Autodesk Inventor part; units mm, degrees
(part 2 of 3)
  spline S130 degree 2 poles (57.6715, -7.9736) (57.2251, -7.5754) (56.7568, -7.4309) knots 0 0 0 1 1 1
  line L163 (56.7568, -7.4309) -> (56.735, -7.3434)
  spline S131 degree 2 poles (56.735, -7.3434) (56.8662, -7.2603) (56.9144, -7.1727) knots 0 0 0 1 1 1
  spline S132 degree 2 poles (56.9144, -7.1727) (57.0019, -7.024) (57.0019, -6.8139) knots 0 0 0 1 1 1
  line L164 (57.0019, -6.8139) -> (57.0019, -4.7133)
  line L165 (57.0019, -4.7133) -> (56.6649, -4.7133)
  line L166 (56.6649, -4.7133) -> (56.6649, -4.3107)
  line L167 (56.6649, -4.3107) -> (57.0019, -4.3107)
  line L168 (57.0019, -4.3107) -> (57.0019, -3.4443)
  spline S133 degree 2 poles (57.0019, -3.4443) (57.5402, -3.0767) (57.8159, -2.8272) knots 0 0 0 1 1 1
  line L169 (57.8159, -2.8272) -> (58.4985, -2.9979)
  line L170 (58.7611, -4.5383) -> (59.7589, -3.3042)
  line L171 (59.7589, -3.3042) -> (59.8639, -3.3042)
  line L172 (59.8639, -3.3042) -> (59.8289, -4.2932)
  line L173 (59.8289, -4.2932) -> (60.551, -4.2932)
  line L174 (60.551, -4.2932) -> (60.551, -4.6958)
  line L175 (60.551, -4.6958) -> (59.8289, -4.6958)
  line L176 (59.8289, -4.6958) -> (59.8289, -7.1159)
  line L177 (59.8289, -7.1159) -> (60.2315, -7.4134)
  line L178 (60.2315, -7.4134) -> (60.4634, -7.234)
  line L179 (60.4634, -7.234) -> (60.5553, -7.3434)
  line L180 (60.5553, -7.3434) -> (59.7633, -7.9736)
  spline S134 degree 2 poles (59.7633, -7.9736) (59.3563, -7.5622) (58.8486, -7.4134) knots 0 0 0 1 1 1
  line L181 (58.8486, -7.4134) -> (58.8486, -7.3434)
  spline S135 degree 2 poles (58.8486, -7.3434) (58.9931, -7.2471) (59.0368, -7.1421) knots 0 0 0 1 1 1
  spline S136 degree 2 poles (59.0368, -7.1421) (59.0981, -7.0108) (59.0981, -6.757) knots 0 0 0 1 1 1
  line L182 (59.0981, -6.757) -> (59.0981, -4.6958)
  line L183 (59.0981, -4.6958) -> (58.7611, -4.6958)
  line L184 (58.7611, -4.6958) -> (58.7611, -4.5383)
  point P0 (76.2, -5.7603)
  point P1 (0, 5.7603)
  constraints: 2 other
extrude "Extrusion5" add sketch "Sketch6" along normal blind 0.2286
sketch "Sketch7" plane through (-5.7603, -3.3257, 0) normal (-0.8660254, 0.5, 0) x (0, 0, 1)
  line L0 (0.5735, 1.7459) -> (40.1435, 1.7459) construction
  line L1 (40.1435, 1.7459) -> (40.1435, 0.1688) construction
  line L2 (40.1435, 0.1688) -> (0.5735, 0.1688) construction
  line L3 (0.5735, 0.1688) -> (0.5735, 1.7459) construction
  spline S0 degree 2 poles (2.0565, 0.9853) (2.0565, 0.867) (1.9917, 0.6457) (1.931, 0.5541) knots 0 0 0 1 2 2 2
  line L4 (1.931, 0.5541) -> (1.5728, 0.5541)
  line L5 (1.5728, 0.5541) -> (1.5512, 0.6529)
  spline S1 degree 2 poles (1.5512, 0.6529) (1.4936, 0.6045) (1.3978, 0.5469) (1.3145, 0.5469) knots 0 0 0 1 2 2 2
  spline S2 degree 2 poles (1.3145, 0.5469) (1.1838, 0.5469) (1.016, 0.7579) (1.016, 0.9576) knots 0 0 0 1 2 2 2
  spline S3 degree 2 poles (1.016, 0.9576) (1.016, 1.1582) (1.2219, 1.3816) (1.3546, 1.3816) knots 0 0 0 1 2 2 2
  spline S4 degree 2 poles (1.3546, 1.3816) (1.4164, 1.3816) (1.5049, 1.3507) (1.5502, 1.325) knots 0 0 0 1 2 2 2
  line L6 (1.5502, 1.325) -> (1.5502, 1.3661)
  line L7 (1.5502, 1.3661) -> (1.685, 1.3661)
  line L8 (1.685, 1.3661) -> (1.685, 0.6488)
  line L9 (1.685, 0.6488) -> (1.8785, 0.6488)
  spline S5 degree 2 poles (1.8785, 0.6488) (1.9114, 0.7095) (1.9392, 0.902) (1.9392, 0.9802) knots 0 0 0 1 2 2 2
  spline S6 degree 2 poles (1.9392, 0.9802) (1.9392, 1.2591) (1.6551, 1.5987) (1.3886, 1.5987) knots 0 0 0 1 2 2 2
  spline S7 degree 2 poles (1.3886, 1.5987) (1.1364, 1.5987) (0.8081, 1.2313) (0.8081, 0.9689) knots 0 0 0 1 2 2 2
  spline S8 degree 2 poles (0.8081, 0.9689) (0.8081, 0.6879) (1.1272, 0.339) (1.3845, 0.339) knots 0 0 0 1 2 2 2
  spline S9 degree 2 poles (1.3845, 0.339) (1.4534, 0.339) (1.6068, 0.3575) (1.6747, 0.3781) knots 0 0 0 1 2 2 2
  line L10 (1.6747, 0.3781) -> (1.6747, 0.2577)
  spline S10 degree 2 poles (1.6747, 0.2577) (1.6027, 0.2402) (1.4555, 0.2268) (1.3834, 0.2268) knots 0 0 0 1 2 2 2
  spline S11 degree 2 poles (1.3834, 0.2268) (1.0819, 0.2268) (0.6857, 0.6416) (0.6857, 0.9709) knots 0 0 0 1 2 2 2
  spline S12 degree 2 poles (0.6857, 0.9709) (0.6857, 1.2838) (1.0942, 1.714) (1.3876, 1.714) knots 0 0 0 1 2 2 2
  spline S13 degree 2 poles (1.3876, 1.714) (1.7015, 1.714) (2.0565, 1.3095) (2.0565, 0.9853) knots 0 0 0 1 2 2 2
  line L11 (1.5481, 0.7672) -> (1.5481, 1.2087)
  spline S14 degree 2 poles (1.5481, 1.2087) (1.5008, 1.2334) (1.4205, 1.255) (1.3762, 1.255) knots 0 0 0 1 2 2 2
  spline S15 degree 2 poles (1.3762, 1.255) (1.2795, 1.255) (1.1622, 1.1109) (1.1622, 0.9596) knots 0 0 0 1 2 2 2
  spline S16 degree 2 poles (1.1622, 0.9596) (1.1622, 0.8238) (1.2507, 0.6786) (1.3484, 0.6786) knots 0 0 0 1 2 2 2
  spline S17 degree 2 poles (1.3484, 0.6786) (1.3999, 0.6786) (1.5018, 0.728) (1.5481, 0.7672) knots 0 0 0 1 2 2 2
  line L12 (3.379, 0.4193) -> (3.2102, 0.4193)
  line L13 (3.2102, 0.4193) -> (3.2102, 1.5133)
  line L14 (3.2102, 1.5133) -> (2.8788, 0.7692)
  line L15 (2.8788, 0.7692) -> (2.7759, 0.7692)
  line L16 (2.7759, 0.7692) -> (2.4476, 1.5133)
  line L17 (2.4476, 1.5133) -> (2.4476, 0.4193)
  line L18 (2.4476, 0.4193) -> (2.2901, 0.4193)
  line L19 (2.2901, 0.4193) -> (2.2901, 1.6893)
  line L20 (2.2901, 1.6893) -> (2.5207, 1.6893)
  line L21 (2.5207, 1.6893) -> (2.8377, 0.9823)
  line L22 (2.8377, 0.9823) -> (3.1444, 1.6893)
  line L23 (3.1444, 1.6893) -> (3.379, 1.6893)
  line L24 (3.379, 1.6893) -> (3.379, 0.4193)
  line L25 (3.7876, 0.4193) -> (3.627, 0.4193)
  line L26 (3.627, 0.4193) -> (3.627, 1.3723)
  line L27 (3.627, 1.3723) -> (3.7876, 1.3723)
  line L28 (3.7876, 1.3723) -> (3.7876, 0.4193)
  line L29 (3.7989, 1.5308) -> (3.6167, 1.5308)
  line L30 (3.6167, 1.5308) -> (3.6167, 1.6975)
  line L31 (3.6167, 1.6975) -> (3.7989, 1.6975)
  line L32 (3.7989, 1.6975) -> (3.7989, 1.5308)
  spline S18 degree 2 poles (4.2806, 0.3967) (4.1848, 0.3967) (4.0192, 0.4481) (3.9646, 0.4769) knots 0 0 0 1 2 2 2
  line L33 (3.9646, 0.4769) -> (3.9646, 0.657)
  line L34 (3.9646, 0.657) -> (3.9728, 0.657)
  spline S19 degree 2 poles (3.9728, 0.657) (3.9934, 0.6406) (4.049, 0.6015) (4.0953, 0.5798) knots 0 0 0 1 2 2 2
  spline S20 degree 2 poles (4.0953, 0.5798) (4.1354, 0.5603) (4.2342, 0.5315) (4.2867, 0.5315) knots 0 0 0 1 2 2 2
  spline S21 degree 2 poles (4.2867, 0.5315) (4.3248, 0.5315) (4.4123, 0.549) (4.4329, 0.5634) knots 0 0 0 1 2 2 2
  spline S22 degree 2 poles (4.4329, 0.5634) (4.4627, 0.5829) (4.4895, 0.6272) (4.4895, 0.6725) knots 0 0 0 1 2 2 2
  spline S23 degree 2 poles (4.4895, 0.6725) (4.4895, 0.7291) (4.4277, 0.7877) (4.3485, 0.8073) knots 0 0 0 1 2 2 2
  spline S24 degree 2 poles (4.3485, 0.8073) (4.3176, 0.8145) (4.2188, 0.8351) (4.1766, 0.8464) knots 0 0 0 1 2 2 2
  spline S25 degree 2 poles (4.1766, 0.8464) (4.0675, 0.8783) (3.9687, 1.01) (3.9687, 1.1037) knots 0 0 0 1 2 2 2
  spline S26 degree 2 poles (3.9687, 1.1037) (3.9687, 1.2334) (4.1632, 1.395) (4.3238, 1.395) knots 0 0 0 1 2 2 2
  spline S27 degree 2 poles (4.3238, 1.395) (4.403, 1.395) (4.5636, 1.3558) (4.6181, 1.326) knots 0 0 0 1 2 2 2
  line L35 (4.6181, 1.326) -> (4.6181, 1.1541)
  line L36 (4.6181, 1.1541) -> (4.6099, 1.1541)
  spline S28 degree 2 poles (4.6099, 1.1541) (4.5481, 1.2035) (4.3979, 1.2601) (4.3207, 1.2601) knots 0 0 0 1 2 2 2
  spline S29 degree 2 poles (4.3207, 1.2601) (4.2415, 1.2601) (4.1324, 1.1932) (4.1324, 1.1263) knots 0 0 0 1 2 2 2
  spline S30 degree 2 poles (4.1324, 1.1263) (4.1324, 1.0656) (4.1972, 1.007) (4.2692, 0.9884) knots 0 0 0 1 2 2 2
  spline S31 degree 2 poles (4.2692, 0.9884) (4.3042, 0.9792) (4.3927, 0.9606) (4.4411, 0.9493) knots 0 0 0 1 2 2 2
  spline S32 degree 2 poles (4.4411, 0.9493) (4.5461, 0.9226) (4.6531, 0.8001) (4.6531, 0.6941) knots 0 0 0 1 2 2 2
  spline S33 degree 2 poles (4.6531, 0.6941) (4.6531, 0.6323) (4.6048, 0.5232) (4.5574, 0.4831) knots 0 0 0 1 2 2 2
  spline S34 degree 2 poles (4.5574, 0.4831) (4.507, 0.4409) (4.3783, 0.3967) (4.2806, 0.3967) knots 0 0 0 1 2 2 2
  spline S35 degree 2 poles (5.0596, 0.3967) (4.9639, 0.3967) (4.7982, 0.4481) (4.7437, 0.4769) knots 0 0 0 1 2 2 2
  line L37 (4.7437, 0.4769) -> (4.7437, 0.657)
  line L38 (4.7437, 0.657) -> (4.7519, 0.657)
  spline S36 degree 2 poles (4.7519, 0.657) (4.7725, 0.6406) (4.8281, 0.6015) (4.8744, 0.5798) knots 0 0 0 1 2 2 2
  spline S37 degree 2 poles (4.8744, 0.5798) (4.9145, 0.5603) (5.0133, 0.5315) (5.0658, 0.5315) knots 0 0 0 1 2 2 2
  spline S38 degree 2 poles (5.0658, 0.5315) (5.1039, 0.5315) (5.1914, 0.549) (5.212, 0.5634) knots 0 0 0 1 2 2 2
  spline S39 degree 2 poles (5.212, 0.5634) (5.2418, 0.5829) (5.2686, 0.6272) (5.2686, 0.6725) knots 0 0 0 1 2 2 2
  spline S40 degree 2 poles (5.2686, 0.6725) (5.2686, 0.7291) (5.2068, 0.7877) (5.1276, 0.8073) knots 0 0 0 1 2 2 2
  spline S41 degree 2 poles (5.1276, 0.8073) (5.0967, 0.8145) (4.9979, 0.8351) (4.9557, 0.8464) knots 0 0 0 1 2 2 2
  spline S42 degree 2 poles (4.9557, 0.8464) (4.8466, 0.8783) (4.7478, 1.01) (4.7478, 1.1037) knots 0 0 0 1 2 2 2
  spline S43 degree 2 poles (4.7478, 1.1037) (4.7478, 1.2334) (4.9423, 1.395) (5.1029, 1.395) knots 0 0 0 1 2 2 2
  spline S44 degree 2 poles (5.1029, 1.395) (5.1821, 1.395) (5.3427, 1.3558) (5.3972, 1.326) knots 0 0 0 1 2 2 2
  line L39 (5.3972, 1.326) -> (5.3972, 1.1541)
  line L40 (5.3972, 1.1541) -> (5.389, 1.1541)
  spline S45 degree 2 poles (5.389, 1.1541) (5.3272, 1.2035) (5.177, 1.2601) (5.0998, 1.2601) knots 0 0 0 1 2 2 2
  spline S46 degree 2 poles (5.0998, 1.2601) (5.0205, 1.2601) (4.9114, 1.1932) (4.9114, 1.1263) knots 0 0 0 1 2 2 2
  spline S47 degree 2 poles (4.9114, 1.1263) (4.9114, 1.0656) (4.9763, 1.007) (5.0483, 0.9884) knots 0 0 0 1 2 2 2
  spline S48 degree 2 poles (5.0483, 0.9884) (5.0833, 0.9792) (5.1718, 0.9606) (5.2202, 0.9493) knots 0 0 0 1 2 2 2
  spline S49 degree 2 poles (5.2202, 0.9493) (5.3252, 0.9226) (5.4322, 0.8001) (5.4322, 0.6941) knots 0 0 0 1 2 2 2
  spline S50 degree 2 poles (5.4322, 0.6941) (5.4322, 0.6323) (5.3838, 0.5232) (5.3365, 0.4831) knots 0 0 0 1 2 2 2
  spline S51 degree 2 poles (5.3365, 0.4831) (5.2861, 0.4409) (5.1574, 0.3967) (5.0596, 0.3967) knots 0 0 0 1 2 2 2
  line L41 (5.7451, 0.4193) -> (5.5845, 0.4193)
  line L42 (5.5845, 0.4193) -> (5.5845, 1.3723)
  line L43 (5.5845, 1.3723) -> (5.7451, 1.3723)
  line L44 (5.7451, 1.3723) -> (5.7451, 0.4193)
  line L45 (5.7564, 1.5308) -> (5.5742, 1.5308)
  line L46 (5.5742, 1.5308) -> (5.5742, 1.6975)
  line L47 (5.5742, 1.6975) -> (5.7564, 1.6975)
  line L48 (5.7564, 1.6975) -> (5.7564, 1.5308)
  spline S52 degree 2 poles (6.764, 0.8958) (6.764, 0.655) (6.5324, 0.3925) (6.3389, 0.3925) knots 0 0 0 1 2 2 2
  spline S53 degree 2 poles (6.3389, 0.3925) (6.1403, 0.3925) (5.9128, 0.6632) (5.9128, 0.8958) knots 0 0 0 1 2 2 2
  spline S54 degree 2 poles (5.9128, 0.8958) (5.9128, 1.1346) (6.1475, 1.3991) (6.3389, 1.3991) knots 0 0 0 1 2 2 2
  spline S55 degree 2 poles (6.3389, 1.3991) (6.5324, 1.3991) (6.764, 1.1356) (6.764, 0.8958) knots 0 0 0 1 2 2 2
  spline S56 degree 2 poles (6.5983, 0.8958) (6.5983, 1.0811) (6.4634, 1.2612) (6.3389, 1.2612) knots 0 0 0 1 2 2 2
  spline S57 degree 2 poles (6.3389, 1.2612) (6.2144, 1.2612) (6.0785, 1.0811) (6.0785, 0.8958) knots 0 0 0 1 2 2 2
  spline S58 degree 2 poles (6.0785, 0.8958) (6.0785, 0.7157) (6.2144, 0.5304) (6.3389, 0.5304) knots 0 0 0 1 2 2 2
  spline S59 degree 2 poles (6.3389, 0.5304) (6.4624, 0.5304) (6.5983, 0.7126) (6.5983, 0.8958) knots 0 0 0 1 2 2 2
  line L49 (7.6768, 0.4193) -> (7.5163, 0.4193)
  line L50 (7.5163, 0.4193) -> (7.5163, 0.9627)
  spline S60 degree 2 poles (7.5163, 0.9627) (7.5163, 1.0286) (7.5039, 1.1418) (7.4854, 1.1757) knots 0 0 0 1 2 2 2
  spline S61 degree 2 poles (7.4854, 1.1757) (7.4659, 1.2118) (7.3959, 1.2468) (7.3362, 1.2468) knots 0 0 0 1 2 2 2
  spline S62 degree 2 poles (7.3362, 1.2468) (7.2765, 1.2468) (7.1499, 1.1829) (7.0892, 1.1315) knots 0 0 0 1 2 2 2
  line L51 (7.0892, 1.1315) -> (7.0892, 0.4193)
  line L52 (7.0892, 0.4193) -> (6.9286, 0.4193)
  line L53 (6.9286, 0.4193) -> (6.9286, 1.3723)
  line L54 (6.9286, 1.3723) -> (7.0892, 1.3723)
  line L55 (7.0892, 1.3723) -> (7.0892, 1.2663)
  spline S63 degree 2 poles (7.0892, 1.2663) (7.1612, 1.3311) (7.3002, 1.3991) (7.3784, 1.3991) knots 0 0 0 1 2 2 2
  spline S64 degree 2 poles (7.3784, 1.3991) (7.5183, 1.3991) (7.6768, 1.2138) (7.6768, 1.0378) knots 0 0 0 1 2 2 2
  line L56 (7.6768, 1.0378) -> (7.6768, 0.4193)
  spline S65 degree 2 poles (8.8141, 0.3967) (8.6762, 0.3967) (8.4827, 0.4543) (8.3973, 0.4955) knots 0 0 0 1 2 2 2
  line L57 (8.3973, 0.4955) -> (8.3973, 0.7075)
  line L58 (8.3973, 0.7075) -> (8.4096, 0.7075)
  spline S66 degree 2 poles (8.4096, 0.7075) (8.493, 0.6292) (8.7039, 0.5428) (8.8017, 0.5428) knots 0 0 0 1 2 2 2
  spline S67 degree 2 poles (8.8017, 0.5428) (8.9417, 0.5428) (9.0847, 0.6591) (9.0847, 0.7548) knots 0 0 0 1 2 2 2
  spline S68 degree 2 poles (9.0847, 0.7548) (9.0847, 0.831) (9.0096, 0.9257) (8.9283, 0.9493) knots 0 0 0 1 2 2 2
  spline S69 degree 2 poles (8.9283, 0.9493) (8.8696, 0.9658) (8.7719, 0.9884) (8.6988, 1.007) knots 0 0 0 1 2 2 2
  spline S70 degree 2 poles (8.6988, 1.007) (8.6329, 1.0245) (8.529, 1.0769) (8.4889, 1.1191) knots 0 0 0 1 2 2 2
  spline S71 degree 2 poles (8.4889, 1.1191) (8.4497, 1.1613) (8.4065, 1.2745) (8.4065, 1.3486) knots 0 0 0 1 2 2 2
  spline S72 degree 2 poles (8.4065, 1.3486) (8.4065, 1.503) (8.6473, 1.7119) (8.8336, 1.7119) knots 0 0 0 1 2 2 2
  spline S73 degree 2 poles (8.8336, 1.7119) (8.9407, 1.7119) (9.13, 1.6697) (9.2113, 1.6296) knots 0 0 0 1 2 2 2
  line L59 (9.2113, 1.6296) -> (9.2113, 1.4279)
  line L60 (9.2113, 1.4279) -> (9.199, 1.4279)
  spline S74 degree 2 poles (9.199, 1.4279) (9.1383, 1.4835) (8.9489, 1.5658) (8.8449, 1.5658) knots 0 0 0 1 2 2 2
  spline S75 degree 2 poles (8.8449, 1.5658) (8.7276, 1.5658) (8.5825, 1.4557) (8.5825, 1.3661) knots 0 0 0 1 2 2 2
  spline S76 degree 2 poles (8.5825, 1.3661) (8.5825, 1.2859) (8.6679, 1.1901) (8.7482, 1.1685) knots 0 0 0 1 2 2 2
  spline S77 degree 2 poles (8.7482, 1.1685) (8.8017, 1.1541) (8.9571, 1.1171) (9.0086, 1.1016) knots 0 0 0 1 2 2 2
  spline S78 degree 2 poles (9.0086, 1.1016) (9.1393, 1.0615) (9.2607, 0.8999) (9.2607, 0.7816) knots 0 0 0 1 2 2 2
  spline S79 degree 2 poles (9.2607, 0.7816) (9.2607, 0.7064) (9.2, 0.5624) (9.1455, 0.5119) knots 0 0 0 1 2 2 2
  spline S80 degree 2 poles (9.1455, 0.5119) (9.0847, 0.4563) (8.9304, 0.3967) (8.8141, 0.3967) knots 0 0 0 1 2 2 2
  spline S81 degree 2 poles (9.9513, 0.5202) (9.9318, 0.5057) (9.8659, 0.4543) (9.835, 0.4389) knots 0 0 0 1 2 2 2
  spline S82 degree 2 poles (9.835, 0.4389) (9.7928, 0.4162) (9.7136, 0.3925) (9.6415, 0.3925) knots 0 0 0 1 2 2 2
  spline S83 degree 2 poles (9.6415, 0.3925) (9.5829, 0.3925) (9.4769, 0.4368) (9.4367, 0.4769) knots 0 0 0 1 2 2 2
  spline S84 degree 2 poles (9.4367, 0.4769) (9.3986, 0.516) (9.3523, 0.6313) (9.3523, 0.6951) knots 0 0 0 1 2 2 2
  spline S85 degree 2 poles (9.3523, 0.6951) (9.3523, 0.7939) (9.4357, 0.9339) (9.5263, 0.974) knots 0 0 0 1 2 2 2
  spline S86 degree 2 poles (9.5263, 0.974) (9.6065, 1.0111) (9.8247, 1.0389) (9.9513, 1.0461) knots 0 0 0 1 2 2 2
  line L61 (9.9513, 1.0461) -> (9.9513, 1.0769)
  spline S87 degree 2 poles (9.9513, 1.0769) (9.9513, 1.1325) (9.9173, 1.2015) (9.8865, 1.221) knots 0 0 0 1 2 2 2
  spline S88 degree 2 poles (9.8865, 1.221) (9.8556, 1.2406) (9.7671, 1.2529) (9.7197, 1.2529) knots 0 0 0 1 2 2 2
  spline S89 degree 2 poles (9.7197, 1.2529) (9.6642, 1.2529) (9.5139, 1.22) (9.4388, 1.1881) knots 0 0 0 1 2 2 2
  line L62 (9.4388, 1.1881) -> (9.4295, 1.1881)
  line L63 (9.4295, 1.1881) -> (9.4295, 1.3517)
  spline S90 degree 2 poles (9.4295, 1.3517) (9.4738, 1.3641) (9.6395, 1.395) (9.7208, 1.395) knots 0 0 0 1 2 2 2
  spline S91 degree 2 poles (9.7208, 1.395) (9.8196, 1.395) (9.9544, 1.3641) (10.0079, 1.3239) knots 0 0 0 1 2 2 2
  spline S92 degree 2 poles (10.0079, 1.3239) (10.0604, 1.2848) (10.1119, 1.1603) (10.1119, 1.0708) knots 0 0 0 1 2 2 2
  line L64 (10.1119, 1.0708) -> (10.1119, 0.4193)
  line L65 (10.1119, 0.4193) -> (9.9513, 0.4193)
  line L66 (9.9513, 0.4193) -> (9.9513, 0.5202)
  line L67 (9.9513, 0.6539) -> (9.9513, 0.9184)
  spline S93 degree 2 poles (9.9513, 0.9184) (9.8937, 0.9133) (9.7197, 0.8958) (9.6652, 0.8793) knots 0 0 0 1 2 2 2
  spline S94 degree 2 poles (9.6652, 0.8793) (9.6014, 0.8598) (9.518, 0.7785) (9.518, 0.7064) knots 0 0 0 1 2 2 2
  spline S95 degree 2 poles (9.518, 0.7064) (9.518, 0.6241) (9.6107, 0.5407) (9.6992, 0.5407) knots 0 0 0 1 2 2 2
  spline S96 degree 2 poles (9.6992, 0.5407) (9.7743, 0.5407) (9.8978, 0.6056) (9.9513, 0.6539) knots 0 0 0 1 2 2 2
  line L68 (11.0855, 0.4193) -> (10.9249, 0.4193)
  line L69 (10.9249, 0.4193) -> (10.9249, 0.9627)
  spline S97 degree 2 poles (10.9249, 0.9627) (10.9249, 1.0286) (10.9126, 1.1418) (10.894, 1.1757) knots 0 0 0 1 2 2 2
  spline S98 degree 2 poles (10.894, 1.1757) (10.8745, 1.2118) (10.8045, 1.2468) (10.7448, 1.2468) knots 0 0 0 1 2 2 2
  spline S99 degree 2 poles (10.7448, 1.2468) (10.6851, 1.2468) (10.5585, 1.1829) (10.4978, 1.1315) knots 0 0 0 1 2 2 2
  line L70 (10.4978, 1.1315) -> (10.4978, 0.4193)
  line L71 (10.4978, 0.4193) -> (10.3372, 0.4193)
  line L72 (10.3372, 0.4193) -> (10.3372, 1.3723)
  line L73 (10.3372, 1.3723) -> (10.4978, 1.3723)
  line L74 (10.4978, 1.3723) -> (10.4978, 1.2663)
  spline S100 degree 2 poles (10.4978, 1.2663) (10.5698, 1.3311) (10.7088, 1.3991) (10.787, 1.3991) knots 0 0 0 1 2 2 2
  spline S101 degree 2 poles (10.787, 1.3991) (10.927, 1.3991) (11.0855, 1.2138) (11.0855, 1.0378) knots 0 0 0 1 2 2 2
  line L75 (11.0855, 1.0378) -> (11.0855, 0.4193)
  spline S102 degree 2 poles (12.3472, 0.7497) (12.3472, 0.5829) (12.1434, 0.4018) (11.9716, 0.4018) knots 0 0 0 1 2 2 2
  spline S103 degree 2 poles (11.9716, 0.4018) (11.9304, 0.4018) (11.7935, 0.4162) (11.7472, 0.4265) knots 0 0 0 1 2 2 2
  line L76 (11.7472, 0.4265) -> (11.7472, 0.5891)
  line L77 (11.7472, 0.5891) -> (11.7565, 0.5891)
  spline S104 degree 2 poles (11.7565, 0.5891) (11.7915, 0.5768) (11.8954, 0.5479) (11.9489, 0.5479) knots 0 0 0 1 2 2 2
  spline S105 degree 2 poles (11.9489, 0.5479) (12.0272, 0.5479) (12.1208, 0.584) (12.1424, 0.6169) knots 0 0 0 1 2 2 2
  spline S106 degree 2 poles (12.1424, 0.6169) (12.1661, 0.6509) (12.1784, 0.7497) (12.1784, 0.8145) knots 0 0 0 1 2 2 2
  line L78 (12.1784, 0.8145) -> (12.1784, 1.5545)
  line L79 (12.1784, 1.5545) -> (11.9098, 1.5545)
  line L80 (11.9098, 1.5545) -> (11.9098, 1.6893)
  line L81 (11.9098, 1.6893) -> (12.3472, 1.6893)
  line L82 (12.3472, 1.6893) -> (12.3472, 0.7497)
  spline S107 degree 2 poles (13.3671, 0.8958) (13.3671, 0.655) (13.1356, 0.3925) (12.9421, 0.3925) knots 0 0 0 1 2 2 2
  spline S108 degree 2 poles (12.9421, 0.3925) (12.7435, 0.3925) (12.516, 0.6632) (12.516, 0.8958) knots 0 0 0 1 2 2 2
  spline S109 degree 2 poles (12.516, 0.8958) (12.516, 1.1346) (12.7507, 1.3991) (12.9421, 1.3991) knots 0 0 0 1 2 2 2
  spline S110 degree 2 poles (12.9421, 1.3991) (13.1356, 1.3991) (13.3671, 1.1356) (13.3671, 0.8958) knots 0 0 0 1 2 2 2
  spline S111 degree 2 poles (13.2014, 0.8958) (13.2014, 1.0811) (13.0666, 1.2612) (12.9421, 1.2612) knots 0 0 0 1 2 2 2
  spline S112 degree 2 poles (12.9421, 1.2612) (12.8176, 1.2612) (12.6817, 1.0811) (12.6817, 0.8958) knots 0 0 0 1 2 2 2
  spline S113 degree 2 poles (12.6817, 0.8958) (12.6817, 0.7157) (12.8176, 0.5304) (12.9421, 0.5304) knots 0 0 0 1 2 2 2
  spline S114 degree 2 poles (12.9421, 0.5304) (13.0656, 0.5304) (13.2014, 0.7126) (13.2014, 0.8958) knots 0 0 0 1 2 2 2
  spline S115 degree 2 poles (13.7891, 0.3967) (13.6934, 0.3967) (13.5277, 0.4481) (13.4731, 0.4769) knots 0 0 0 1 2 2 2
  line L83 (13.4731, 0.4769) -> (13.4731, 0.657)
  line L84 (13.4731, 0.657) -> (13.4814, 0.657)
  spline S116 degree 2 poles (13.4814, 0.657) (13.502, 0.6406) (13.5575, 0.6015) (13.6038, 0.5798) knots 0 0 0 1 2 2 2
  spline S117 degree 2 poles (13.6038, 0.5798) (13.644, 0.5603) (13.7428, 0.5315) (13.7953, 0.5315) knots 0 0 0 1 2 2 2
  spline S118 degree 2 poles (13.7953, 0.5315) (13.8334, 0.5315) (13.9208, 0.549) (13.9414, 0.5634) knots 0 0 0 1 2 2 2
  spline S119 degree 2 poles (13.9414, 0.5634) (13.9713, 0.5829) (13.998, 0.6272) (13.998, 0.6725) knots 0 0 0 1 2 2 2
  spline S120 degree 2 poles (13.998, 0.6725) (13.998, 0.7291) (13.9363, 0.7877) (13.857, 0.8073) knots 0 0 0 1 2 2 2
  spline S121 degree 2 poles (13.857, 0.8073) (13.8261, 0.8145) (13.7273, 0.8351) (13.6851, 0.8464) knots 0 0 0 1 2 2 2
  spline S122 degree 2 poles (13.6851, 0.8464) (13.5761, 0.8783) (13.4773, 1.01) (13.4773, 1.1037) knots 0 0 0 1 2 2 2
  spline S123 degree 2 poles (13.4773, 1.1037) (13.4773, 1.2334) (13.6718, 1.395) (13.8323, 1.395) knots 0 0 0 1 2 2 2
  spline S124 degree 2 poles (13.8323, 1.395) (13.9116, 1.395) (14.0721, 1.3558) (14.1267, 1.326) knots 0 0 0 1 2 2 2
  line L85 (14.1267, 1.326) -> (14.1267, 1.1541)
  line L86 (14.1267, 1.1541) -> (14.1184, 1.1541)
  spline S125 degree 2 poles (14.1184, 1.1541) (14.0567, 1.2035) (13.9064, 1.2601) (13.8292, 1.2601) knots 0 0 0 1 2 2 2
  spline S126 degree 2 poles (13.8292, 1.2601) (13.75, 1.2601) (13.6409, 1.1932) (13.6409, 1.1263) knots 0 0 0 1 2 2 2
  spline S127 degree 2 poles (13.6409, 1.1263) (13.6409, 1.0656) (13.7057, 1.007) (13.7778, 0.9884) knots 0 0 0 1 2 2 2
  spline S128 degree 2 poles (13.7778, 0.9884) (13.8128, 0.9792) (13.9013, 0.9606) (13.9496, 0.9493) knots 0 0 0 1 2 2 2
  spline S129 degree 2 poles (13.9496, 0.9493) (14.0546, 0.9226) (14.1617, 0.8001) (14.1617, 0.6941) knots 0 0 0 1 2 2 2
  spline S130 degree 2 poles (14.1617, 0.6941) (14.1617, 0.6323) (14.1133, 0.5232) (14.0659, 0.4831) knots 0 0 0 1 2 2 2
  spline S131 degree 2 poles (14.0659, 0.4831) (14.0155, 0.4409) (13.8869, 0.3967) (13.7891, 0.3967) knots 0 0 0 1 2 2 2
  spline S132 degree 2 poles (14.7246, 0.3977) (14.4961, 0.3977) (14.245, 0.6539) (14.245, 0.8907) knots 0 0 0 1 2 2 2
  spline S133 degree 2 poles (14.245, 0.8907) (14.245, 1.1233) (14.4889, 1.3991) (14.6855, 1.3991) knots 0 0 0 1 2 2 2
  spline S134 degree 2 poles (14.6855, 1.3991) (14.774, 1.3991) (14.9109, 1.3476) (14.9613, 1.2931) knots 0 0 0 1 2 2 2
  spline S135 degree 2 poles (14.9613, 1.2931) (15.0128, 1.2385) (15.0673, 1.0811) (15.0673, 0.9668) knots 0 0 0 1 2 2 2
  line L87 (15.0673, 0.9668) -> (15.0673, 0.8793)
  line L88 (15.0673, 0.8793) -> (14.4076, 0.8793)
  spline S136 degree 2 poles (14.4076, 0.8793) (14.4076, 0.7136) (14.5744, 0.5377) (14.7226, 0.5377) knots 0 0 0 1 2 2 2
  spline S137 degree 2 poles (14.7226, 0.5377) (14.775, 0.5377) (14.8769, 0.5613) (14.9181, 0.5798) knots 0 0 0 1 2 2 2
  spline S138 degree 2 poles (14.9181, 0.5798) (14.9613, 0.6004) (15.021, 0.6365) (15.0406, 0.6529) knots 0 0 0 1 2 2 2
  line L89 (15.0406, 0.6529) -> (15.0498, 0.6529)
  line L90 (15.0498, 0.6529) -> (15.0498, 0.478)
  spline S139 degree 2 poles (15.0498, 0.478) (15.022, 0.4666) (14.9377, 0.4337) (14.9047, 0.4244) knots 0 0 0 1 2 2 2
  spline S140 degree 2 poles (14.9047, 0.4244) (14.8584, 0.4111) (14.7822, 0.3977) (14.7246, 0.3977) knots 0 0 0 1 2 2 2
  spline S141 degree 2 poles (14.9109, 1.0018) (14.9088, 1.0666) (14.8821, 1.1613) (14.8563, 1.1932) knots 0 0 0 1 2 2 2
  spline S142 degree 2 poles (14.8563, 1.1932) (14.8286, 1.2293) (14.7411, 1.2673) (14.6762, 1.2673) knots 0 0 0 1 2 2 2
  spline S143 degree 2 poles (14.6762, 1.2673) (14.6124, 1.2673) (14.5229, 1.2293) (14.4858, 1.1922) knots 0 0 0 1 2 2 2
  spline S144 degree 2 poles (14.4858, 1.1922) (14.4498, 1.1541) (14.4128, 1.0625) (14.4076, 1.0018) knots 0 0 0 1 2 2 2
  line L91 (14.4076, 1.0018) -> (14.9109, 1.0018)
  line L92 (16.7099, 0.4193) -> (16.5411, 0.4193)
  line L93 (16.5411, 0.4193) -> (16.5411, 1.0409)
  line L94 (16.5411, 1.0409) -> (15.9565, 1.0409)
  line L95 (15.9565, 1.0409) -> (15.9565, 0.4193)
  line L96 (15.9565, 0.4193) -> (15.7878, 0.4193)
  line L97 (15.7878, 0.4193) -> (15.7878, 1.6893)
  line L98 (15.7878, 1.6893) -> (15.9565, 1.6893)
  line L99 (15.9565, 1.6893) -> (15.9565, 1.1912)
  line L100 (15.9565, 1.1912) -> (16.5411, 1.1912)
  line L101 (16.5411, 1.1912) -> (16.5411, 1.6893)
  line L102 (16.5411, 1.6893) -> (16.7099, 1.6893)
  line L103 (16.7099, 1.6893) -> (16.7099, 0.4193)
  line L104 (17.1185, 0.4193) -> (16.9579, 0.4193)
  line L105 (16.9579, 0.4193) -> (16.9579, 1.3723)
  line L106 (16.9579, 1.3723) -> (17.1185, 1.3723)
  line L107 (17.1185, 1.3723) -> (17.1185, 0.4193)
  line L108 (17.1298, 1.5308) -> (16.9476, 1.5308)
  line L109 (16.9476, 1.5308) -> (16.9476, 1.6975)
  line L110 (16.9476, 1.6975) -> (17.1298, 1.6975)
  line L111 (17.1298, 1.6975) -> (17.1298, 1.5308)
  spline S145 degree 2 poles (17.3881, 0.267) (17.4046, 0.2598) (17.4674, 0.2371) (17.5075, 0.2279) knots 0 0 0 1 2 2 2
  spline S146 degree 2 poles (17.5075, 0.2279) (17.5518, 0.2166) (17.6269, 0.2032) (17.6711, 0.2032) knots 0 0 0 1 2 2 2
  spline S147 degree 2 poles (17.6711, 0.2032) (17.7452, 0.2032) (17.8482, 0.2423) (17.877, 0.2773) knots 0 0 0 1 2 2 2
  spline S148 degree 2 poles (17.877, 0.2773) (17.9048, 0.3123) (17.9264, 0.4039) (17.9264, 0.4625) knots 0 0 0 1 2 2 2
  line L112 (17.9264, 0.4625) -> (17.9264, 0.5459)
  spline S149 degree 2 poles (17.9264, 0.5459) (17.8615, 0.4893) (17.737, 0.4358) (17.6434, 0.4358) knots 0 0 0 1 2 2 2
  spline S150 degree 2 poles (17.6434, 0.4358) (17.4807, 0.4358) (17.2883, 0.6776) (17.2883, 0.9051) knots 0 0 0 1 2 2 2
  spline S151 degree 2 poles (17.2883, 0.9051) (17.2883, 1.0234) (17.3552, 1.2066) (17.4108, 1.2715) knots 0 0 0 1 2 2 2
  spline S152 degree 2 poles (17.4108, 1.2715) (17.4643, 1.3322) (17.6114, 1.3991) (17.6897, 1.3991) knots 0 0 0 1 2 2 2
  spline S153 degree 2 poles (17.6897, 1.3991) (17.7638, 1.3991) (17.8718, 1.3641) (17.9264, 1.3322) knots 0 0 0 1 2 2 2
  line L113 (17.9264, 1.3322) -> (17.9356, 1.3723)
  line L114 (17.9356, 1.3723) -> (18.0869, 1.3723)
  line L115 (18.0869, 1.3723) -> (18.0869, 0.5284)
  spline S154 degree 2 poles (18.0869, 0.5284) (18.0869, 0.2855) (17.8759, 0.0591) (17.6588, 0.0591) knots 0 0 0 1 2 2 2
  spline S155 degree 2 poles (17.6588, 0.0591) (17.5888, 0.0591) (17.4427, 0.0817) (17.3799, 0.1003) knots 0 0 0 1 2 2 2
  line L116 (17.3799, 0.1003) -> (17.3799, 0.267)
  line L117 (17.3799, 0.267) -> (17.3881, 0.267)
  line L118 (17.9264, 0.6776) -> (17.9264, 1.2015)
  spline S156 degree 2 poles (17.9264, 1.2015) (17.8667, 1.2303) (17.7658, 1.255) (17.7154, 1.255) knots 0 0 0 1 2 2 2
  spline S157 degree 2 poles (17.7154, 1.255) (17.5939, 1.255) (17.454, 1.0759) (17.454, 0.9082) knots 0 0 0 1 2 2 2
  spline S158 degree 2 poles (17.454, 0.9082) (17.454, 0.7497) (17.56, 0.584) (17.6794, 0.584) knots 0 0 0 1 2 2 2
  spline S159 degree 2 poles (17.6794, 0.584) (17.7422, 0.584) (17.8739, 0.6334) (17.9264, 0.6776) knots 0 0 0 1 2 2 2
  line L119 (19.0677, 0.4193) -> (18.9072, 0.4193)
  line L120 (18.9072, 0.4193) -> (18.9072, 0.9627)
  spline S160 degree 2 poles (18.9072, 0.9627) (18.9072, 1.0286) (18.8948, 1.1418) (18.8763, 1.1757) knots 0 0 0 1 2 2 2
  spline S161 degree 2 poles (18.8763, 1.1757) (18.8567, 1.2118) (18.7868, 1.2468) (18.7271, 1.2468) knots 0 0 0 1 2 2 2
  spline S162 degree 2 poles (18.7271, 1.2468) (18.6674, 1.2468) (18.5408, 1.1829) (18.4801, 1.1315) knots 0 0 0 1 2 2 2
  line L121 (18.4801, 1.1315) -> (18.4801, 0.4193)
  line L122 (18.4801, 0.4193) -> (18.3195, 0.4193)
  line L123 (18.3195, 0.4193) -> (18.3195, 1.7459)
  line L124 (18.3195, 1.7459) -> (18.4801, 1.7459)
  line L125 (18.4801, 1.7459) -> (18.4801, 1.2663)
  spline S163 degree 2 poles (18.4801, 1.2663) (18.5521, 1.3311) (18.691, 1.3991) (18.7693, 1.3991) knots 0 0 0 1 2 2 2
  spline S164 degree 2 poles (18.7693, 1.3991) (18.9092, 1.3991) (19.0677, 1.2138) (19.0677, 1.0378) knots 0 0 0 1 2 2 2
  line L126 (19.0677, 1.0378) -> (19.0677, 0.4193)
  spline S165 degree 2 poles (20.205, 0.3967) (20.0671, 0.3967) (19.8736, 0.4543) (19.7881, 0.4955) knots 0 0 0 1 2 2 2
  line L127 (19.7881, 0.4955) -> (19.7881, 0.7075)
  line L128 (19.7881, 0.7075) -> (19.8005, 0.7075)
  spline S166 degree 2 poles (19.8005, 0.7075) (19.8839, 0.6292) (20.0948, 0.5428) (20.1926, 0.5428) knots 0 0 0 1 2 2 2
  spline S167 degree 2 poles (20.1926, 0.5428) (20.3326, 0.5428) (20.4756, 0.6591) (20.4756, 0.7548) knots 0 0 0 1 2 2 2
  spline S168 degree 2 poles (20.4756, 0.7548) (20.4756, 0.831) (20.4005, 0.9257) (20.3192, 0.9493) knots 0 0 0 1 2 2 2
  spline S169 degree 2 poles (20.3192, 0.9493) (20.2605, 0.9658) (20.1628, 0.9884) (20.0897, 1.007) knots 0 0 0 1 2 2 2
  spline S170 degree 2 poles (20.0897, 1.007) (20.0238, 1.0245) (19.9199, 1.0769) (19.8797, 1.1191) knots 0 0 0 1 2 2 2
  spline S171 degree 2 poles (19.8797, 1.1191) (19.8406, 1.1613) (19.7974, 1.2745) (19.7974, 1.3486) knots 0 0 0 1 2 2 2
  spline S172 degree 2 poles (19.7974, 1.3486) (19.7974, 1.503) (20.0382, 1.7119) (20.2245, 1.7119) knots 0 0 0 1 2 2 2
  spline S173 degree 2 poles (20.2245, 1.7119) (20.3316, 1.7119) (20.5209, 1.6697) (20.6022, 1.6296) knots 0 0 0 1 2 2 2
  line L129 (20.6022, 1.6296) -> (20.6022, 1.4279)
  line L130 (20.6022, 1.4279) -> (20.5899, 1.4279)
  spline S174 degree 2 poles (20.5899, 1.4279) (20.5292, 1.4835) (20.3398, 1.5658) (20.2358, 1.5658) knots 0 0 0 1 2 2 2
  spline S175 degree 2 poles (20.2358, 1.5658) (20.1185, 1.5658) (19.9734, 1.4557) (19.9734, 1.3661) knots 0 0 0 1 2 2 2
  spline S176 degree 2 poles (19.9734, 1.3661) (19.9734, 1.2859) (20.0588, 1.1901) (20.1391, 1.1685) knots 0 0 0 1 2 2 2
  spline S177 degree 2 poles (20.1391, 1.1685) (20.1926, 1.1541) (20.348, 1.1171) (20.3995, 1.1016) knots 0 0 0 1 2 2 2
  spline S178 degree 2 poles (20.3995, 1.1016) (20.5302, 1.0615) (20.6516, 0.8999) (20.6516, 0.7816) knots 0 0 0 1 2 2 2
  spline S179 degree 2 poles (20.6516, 0.7816) (20.6516, 0.7064) (20.5909, 0.5624) (20.5364, 0.5119) knots 0 0 0 1 2 2 2
  spline S180 degree 2 poles (20.5364, 0.5119) (20.4756, 0.4563) (20.3213, 0.3967) (20.205, 0.3967) knots 0 0 0 1 2 2 2
  spline S181 degree 2 poles (21.1899, 0.3977) (21.0911, 0.3977) (20.9274, 0.4584) (20.8688, 0.5202) knots 0 0 0 1 2 2 2
  spline S182 degree 2 poles (20.8688, 0.5202) (20.8101, 0.5809) (20.7453, 0.7682) (20.7453, 0.8937) knots 0 0 0 1 2 2 2
  spline S183 degree 2 poles (20.7453, 0.8937) (20.7453, 1.0193) (20.8122, 1.2025) (20.8688, 1.2642) knots 0 0 0 1 2 2 2
  spline S184 degree 2 poles (20.8688, 1.2642) (20.9254, 1.327) (21.0931, 1.3939) (21.1899, 1.3939) knots 0 0 0 1 2 2 2
  spline S185 degree 2 poles (21.1899, 1.3939) (21.2681, 1.3939) (21.4142, 1.3497) (21.4708, 1.3209) knots 0 0 0 1 2 2 2
  line L131 (21.4708, 1.3209) -> (21.4708, 1.1407)
  line L132 (21.4708, 1.1407) -> (21.4616, 1.1407)
  spline S186 degree 2 poles (21.4616, 1.1407) (21.4441, 1.1552) (21.3906, 1.1922) (21.3525, 1.2118) knots 0 0 0 1 2 2 2
  spline S187 degree 2 poles (21.3525, 1.2118) (21.3185, 1.2282) (21.228, 1.254) (21.1868, 1.254) knots 0 0 0 1 2 2 2
  spline S188 degree 2 poles (21.1868, 1.254) (21.0623, 1.254) (20.911, 1.0656) (20.911, 0.8937) knots 0 0 0 1 2 2 2
  spline S189 degree 2 poles (20.911, 0.8937) (20.911, 0.726) (21.0571, 0.5377) (21.1868, 0.5377) knots 0 0 0 1 2 2 2
  spline S190 degree 2 poles (21.1868, 0.5377) (21.265, 0.5377) (21.407, 0.6025) (21.4616, 0.6529) knots 0 0 0 1 2 2 2
  line L133 (21.4616, 0.6529) -> (21.4708, 0.6529)
  line L134 (21.4708, 0.6529) -> (21.4708, 0.4728)
  spline S191 degree 2 poles (21.4708, 0.4728) (21.4472, 0.4615) (21.3751, 0.4296) (21.3463, 0.4224) knots 0 0 0 1 2 2 2
  spline S192 degree 2 poles (21.3463, 0.4224) (21.3051, 0.41) (21.2403, 0.3977) (21.1899, 0.3977) knots 0 0 0 1 2 2 2
  line L135 (22.3652, 0.4193) -> (22.2046, 0.4193)
  line L136 (22.2046, 0.4193) -> (22.2046, 0.9627)
  spline S193 degree 2 poles (22.2046, 0.9627) (22.2046, 1.0286) (22.1923, 1.1418) (22.1738, 1.1757) knots 0 0 0 1 2 2 2
  spline S194 degree 2 poles (22.1738, 1.1757) (22.1542, 1.2118) (22.0842, 1.2468) (22.0245, 1.2468) knots 0 0 0 1 2 2 2
  spline S195 degree 2 poles (22.0245, 1.2468) (21.9648, 1.2468) (21.8383, 1.1829) (21.7775, 1.1315) knots 0 0 0 1 2 2 2
  line L137 (21.7775, 1.1315) -> (21.7775, 0.4193)
  line L138 (21.7775, 0.4193) -> (21.617, 0.4193)
  line L139 (21.617, 0.4193) -> (21.617, 1.7459)
  line L140 (21.617, 1.7459) -> (21.7775, 1.7459)
  line L141 (21.7775, 1.7459) -> (21.7775, 1.2663)
  spline S196 degree 2 poles (21.7775, 1.2663) (21.8496, 1.3311) (21.9885, 1.3991) (22.0667, 1.3991) knots 0 0 0 1 2 2 2
  spline S197 degree 2 poles (22.0667, 1.3991) (22.2067, 1.3991) (22.3652, 1.2138) (22.3652, 1.0378) knots 0 0 0 1 2 2 2
  line L142 (22.3652, 1.0378) -> (22.3652, 0.4193)
  spline S198 degree 2 poles (23.3738, 0.8958) (23.3738, 0.655) (23.1422, 0.3925) (22.9487, 0.3925) knots 0 0 0 1 2 2 2
  spline S199 degree 2 poles (22.9487, 0.3925) (22.7501, 0.3925) (22.5227, 0.6632) (22.5227, 0.8958) knots 0 0 0 1 2 2 2
  spline S200 degree 2 poles (22.5227, 0.8958) (22.5227, 1.1346) (22.7573, 1.3991) (22.9487, 1.3991) knots 0 0 0 1 2 2 2
  spline S201 degree 2 poles (22.9487, 1.3991) (23.1422, 1.3991) (23.3738, 1.1356) (23.3738, 0.8958) knots 0 0 0 1 2 2 2
  spline S202 degree 2 poles (23.2081, 0.8958) (23.2081, 1.0811) (23.0733, 1.2612) (22.9487, 1.2612) knots 0 0 0 1 2 2 2
  spline S203 degree 2 poles (22.9487, 1.2612) (22.8242, 1.2612) (22.6884, 1.0811) (22.6884, 0.8958) knots 0 0 0 1 2 2 2
  spline S204 degree 2 poles (22.6884, 0.8958) (22.6884, 0.7157) (22.8242, 0.5304) (22.9487, 0.5304) knots 0 0 0 1 2 2 2
  spline S205 degree 2 poles (22.9487, 0.5304) (23.0722, 0.5304) (23.2081, 0.7126) (23.2081, 0.8958) knots 0 0 0 1 2 2 2
  spline S206 degree 2 poles (24.3217, 0.8958) (24.3217, 0.655) (24.0901, 0.3925) (23.8966, 0.3925) knots 0 0 0 1 2 2 2
  spline S207 degree 2 poles (23.8966, 0.3925) (23.698, 0.3925) (23.4705, 0.6632) (23.4705, 0.8958) knots 0 0 0 1 2 2 2
  spline S208 degree 2 poles (23.4705, 0.8958) (23.4705, 1.1346) (23.7052, 1.3991) (23.8966, 1.3991) knots 0 0 0 1 2 2 2
  spline S209 degree 2 poles (23.8966, 1.3991) (24.0901, 1.3991) (24.3217, 1.1356) (24.3217, 0.8958) knots 0 0 0 1 2 2 2
  spline S210 degree 2 poles (24.156, 0.8958) (24.156, 1.0811) (24.0211, 1.2612) (23.8966, 1.2612) knots 0 0 0 1 2 2 2
  spline S211 degree 2 poles (23.8966, 1.2612) (23.7721, 1.2612) (23.6362, 1.0811) (23.6362, 0.8958) knots 0 0 0 1 2 2 2
  spline S212 degree 2 poles (23.6362, 0.8958) (23.6362, 0.7157) (23.7721, 0.5304) (23.8966, 0.5304) knots 0 0 0 1 2 2 2
  spline S213 degree 2 poles (23.8966, 0.5304) (24.0201, 0.5304) (24.156, 0.7126) (24.156, 0.8958) knots 0 0 0 1 2 2 2
  line L143 (24.65, 0.4193) -> (24.4894, 0.4193)
  line L144 (24.4894, 0.4193) -> (24.4894, 1.7459)
  line L145 (24.4894, 1.7459) -> (24.65, 1.7459)
  line L146 (24.65, 1.7459) -> (24.65, 0.4193)
  point P0 (0, 5.7603)
  constraints: 2 other